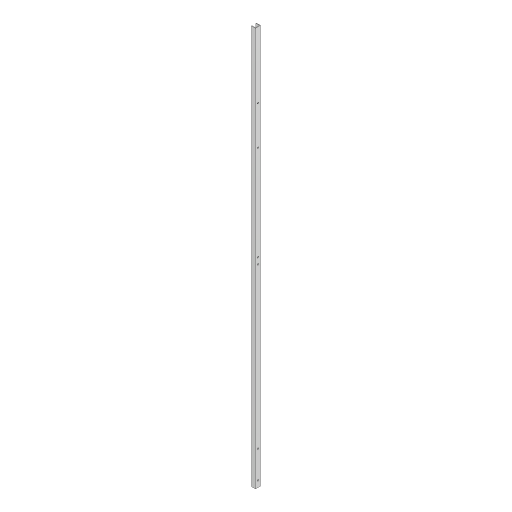
# Autodesk Inventor part: Stringer
Saved by Autodesk Inventor 2024 (Build 280153000, 153)
## iProperties
Created: 2023-12-30
Part Number: Stringer
Material: Aluminum
Document SubType Name: Modeling
Designer: Jamie
Density: 2.7 g/cm^3
Appearance: Satin
Author: Jamie
Autodesk Inventor part; units mm, degrees
ref_plane "YZ Plane" through (0, 0, 0) normal (1, 0, 0) x (0, 1, 0)
ref_plane "XZ Plane" through (0, 0, 0) normal (0, 1, 0) x (-1, 0, 0)
ref_plane "XY Plane" through (0, 0, 0) normal (0, 0, 1) x (1, 0, 0)
sketch "Sketch1" plane through (0, 0, 0) normal (0, 1, 0) x (-1, 0, 0)
  line L0 (0, 0) -> (8, 0)
  line L1 (8, -10) -> (0, -10)
  line L2 (0, -10) -> (0, 0)
  line L3 (8, -1) -> (1, -1)
  line L4 (1, -1) -> (1, -9)
  line L5 (1, -9) -> (8, -9)
  line L6 (8, 0) -> (8, -1)
  line L7 (8, -9) -> (8, -10)
  dimension "d0" = 1
  dimension "d1" = 1
  dimension "d2" = 1
  dimension "d3" = 10
  dimension "d4" = 8
  constraints: 16 end point, 4 parallel, 3 perpendicular, 2 horizontal, 1 collinear
  measures "d0" distance between parallel lines of L3 L0
  measures "d1" distance between parallel lines of L1 L5
  measures "d2" distance between parallel lines of L2 L4
  measures "d3" distance of L1.end L0.start
  measures "d4" distance of L0.start L0.end
extrude "Extrusion1" add sketch "Sketch1" along normal blind 410
sketch "Sketch2" plane through (0, 0, 0) normal (1, 0, 0) x (0, 0, -1)
  line L0 (0, 0) -> (10, 0) projected
  line L1 (0, 0) -> (0, 410) projected
  point P0 (5, 10)
  dimension "d7" = 10
  dimension "d8" = 5
  measures "d7" distance from line of L0 point (5, 10)
  measures "d8" distance from line of L1 point (5, 10)
hole "Hole1" at (0, 10, -5) direction (-1, 0, 0) diameter 3 depth 8 tip angle 118
sketch "Sketch3" plane through (0, 0, 0) normal (1, 0, 0) x (0, 0, -1)
  line L0 (0, 0) -> (0, 410) projected
  line L1 (0, 410) -> (10, 410) projected
  point P0 (5, 277.5)
  point P1 (5, 410)
  dimension "d16" = 5
  dimension "d17" = 132.5
  constraints: 1 midpoint
  measures "d16" distance from line of L0 point (5, 277.5)
  measures "d17" distance of point (5, 410) point (5, 277.5)
hole "Hole2" at (0, 277.5, -5) direction (-1, 0, 0) diameter 3 depth 8 tip angle 118
sketch "Sketch5" plane through (0, 0, 0) normal (1, 0, 0) x (0, 0, -1)
  line L0 (0, 0) -> (0, 410) projected
  circle A0 centre (5, 10) radius 1.5 projected
  point P0 (5, 200)
  dimension "d25" = 5
  dimension "d26" = 190
  measures "d25" distance from line of L0 point (5, 200)
  measures "d26" distance of A0.centre point (5, 200)
hole "Hole3" at (0, 200, -5) direction (-1, 0, 0) diameter 3 depth 8 tip angle 118
sketch "Sketch7" plane through (0, 0, 0) normal (0, -1, 0) x (1, 0, 0)
  line L0 (-8, -9) -> (-1, -9) projected
  line L1 (-8, -9) -> (-1, -9)
  line L2 (-1, -9) -> (-1, -1) projected
  line L3 (-1, -9) -> (-1, -1)
  line L4 (-1, -1) -> (-8, -1) projected
  line L5 (-1, -1) -> (-8, -1)
  line L6 (-8, -1) -> (-8, 0)
  line L7 (-8, 0) -> (0, 0)
  line L8 (0, -10) -> (-8, -10) projected
  line L9 (0, 0) -> (0, -10)
  line L10 (0, -10) -> (-8, -10)
  line L11 (-8, -10) -> (-8, -9)
  constraints: 16 end point, 6 perpendicular, 2 collinear, 1 point on line
extrude "Extrusion2" add sketch "Sketch7" along normal blind 390
sketch "Sketch8" plane through (0, -390, -10) normal (1, 0, 0) x (0, 0, -1)
  line L0 (-10, 0) -> (-10, 800) projected
  circle A0 centre (-5, 400) radius 1.5 projected
  point P0 (-10, 390)
  point P1 (-5, 387.5)
  dimension "d36" = 5
  dimension "d37" = 12.5
  measures "d36" distance from line of L0 point (-5, 387.5)
  measures "d37" distance of A0.centre point (-5, 387.5)
hole "Hole4" at (0, -2.5, -5) direction (-1, 0, 0) diameter 3 depth 16 tip angle 118
sketch "Sketch9" plane through (0, -390, -10) normal (1, 0, 0) x (0, 0, -1)
  line L0 (-10, 0) -> (-10, 800) projected
  line L1 (0, 0) -> (-10, 0) projected
  point P0 (-10, 390)
  point P1 (-5, 12.5)
  dimension "d45" = 5
  dimension "d46" = 12.5
  measures "d45" distance from line of L0 point (-5, 12.5)
  measures "d46" distance from line of L1 point (-5, 12.5)
hole "Hole5" at (0, -377.5, -5) direction (-1, 0, 0) diameter 3 depth 8 tip angle 118
sketch "Sketch10" plane through (0, -390, -10) normal (1, 0, 0) x (0, 0, -1)
  circle A0 centre (-5, 12.5) radius 1.5 projected
  line L0 (-10, 0) -> (-10, 800) projected
  point P0 (-10, 390)
  point P1 (-5, 67.5)
  dimension "d54" = 55
  dimension "d55" = 5
  measures "d54" distance of A0.centre point (-5, 67.5)
  measures "d55" distance from line of L0 point (-5, 67.5)
hole "Hole6" at (0, -322.5, -5) direction (-1, 0, 0) diameter 3 depth 8 tip angle 118
body "Solid1"
